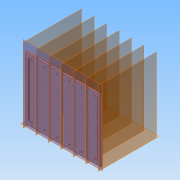
# Autodesk Inventor part: Selection_Ramp 1
Saved by Autodesk Inventor 2018.1 (Build 221171000, 171)
## iProperties
Created: 2019-02-07
Part Number: Selection_Ramp 1
Material: Wood (Oak)
Document SubType Name: Modeling
Designer: James
Density: 0.76 g/cm^3
Appearance: White Oak - Natural Medium Gloss
Author: James
Autodesk Inventor part; units mm, degrees
ref_plane "YZ Plane" through (0, 0, 0) normal (1, 0, 0) x (0, 1, 0)
ref_plane "XZ Plane" through (0, 0, 0) normal (0, 1, 0) x (-1, 0, 0)
ref_plane "XY Plane" through (0, 0, 0) normal (0, 0, 1) x (1, 0, 0)
derived "Prototype_Skeleton.ipt"
ref_plane "Ground" through (0, 0, 0) normal (0, 1, 0) x (-1, 0, 0)
ref_plane "LHS inner" through (0, 0, 0) normal (1, 0, 0) x (0, 1, 0)
ref_plane "RHS inner" through (300, 0, 0) normal (1, 0, 0) x (0, 1, 0)
ref_plane "Lane 1" through (50, 0, 0) normal (1, 0, 0) x (0, 1, 0)
ref_plane "Lane 2" through (100, 0, 0) normal (1, 0, 0) x (0, 1, 0)
ref_plane "Lane 3" through (150, 0, 0) normal (1, 0, 0) x (0, 1, 0)
ref_plane "Lane 4" through (200, 0, 0) normal (1, 0, 0) x (0, 1, 0)
ref_plane "Lane 5" through (250, 0, 0) normal (1, 0, 0) x (0, 1, 0)
ref_plane "Back" through (0, 0, 0) normal (0, 0, 1) x (1, 0, 0)
sketch "Sketch1" plane through (0, 0, 0) normal (0, 1, 0) x (-1, 0, 0)
  line L0 (-300, -50) -> (-300, 300) projected
  line L1 (0, -50) -> (0, 300) projected
  line L2 (-360, 0) -> (60, 0) projected
  line L3 (0, 0) -> (-300, 0)
  line L4 (-300, 0) -> (-300, 250)
  line L5 (-300, 250) -> (0, 250)
  line L6 (0, 250) -> (0, 0)
  dimension "d1" = 250
  constraints: 8 end point, 2 parallel, 1 horizontal, 1 perpendicular, 1 point on line
  measures "d1" distance of L3.end L4.end
extrude "Extrusion1" add sketch "Sketch1" along normal blind 5
sketch "Sketch2" plane through (0, 5, 0) normal (0, 1, 0) x (1, 0, 0)
  line L0 (300, 0) -> (0, 0) projected
  line L1 (0, -250) -> (300, -250) projected
  line L2 (50, 50) -> (50, -300) projected
  point P0 (25, -15)
  point P1 (25, -235)
  dimension "d4" = 15
  dimension "d5" = 15
  dimension "d6" = 220
  dimension "d7" = 25
  constraints: 1 vertical alignment
  measures "d4" distance from line of point (25, -15) L0
  measures "d5" distance from line of L1 point (25, -235)
  measures "d6" distance of point (25, -15) point (25, -235)
  measures "d7" distance from line of L2 point (25, -15)
hole "Hole1" at (25, 5, 15) at (25, 5, 235) direction (0, -1, 0) diameter 4.5 end through all clearance for "Socket Head Cap Screw" size "M4" standard "Ansi Metric M Profile"
pattern_linear "Rectangular Pattern1" count 6 spacing 50 along (1, 0, 0) of "Hole1"
ref_plane "Mid Plane" through (150, 0, 0) normal (-1, 0, 0) x (0, 0, 1)
sketch "Sketch4" plane through (0, 5, 0) normal (0, 1, 0) x (1, 0, 0)
  line L0 (0, 0) -> (0, -250) projected
  line L1 (300, 0) -> (0, 0) projected
  line L2 (0, -250) -> (300, -250) projected
  point P0 (12.5, -167.5)
  point P1 (12.5, -232.5)
  dimension "d29" = 12.5
  dimension "d30" = 65
  dimension "d40" = 17.5
  constraints: 1 vertical alignment
  measures "d29" distance from line of L0 point (12.5, -167.5)
  measures "d30" distance of point (12.5, -167.5) point (12.5, -232.5)
  measures "d40" distance from line of L2 point (12.5, -232.5)
hole "Hole3" at (12.5, 5, 167.5) at (12.5, 5, 232.5) direction (0, -1, 0) diameter 4.5 end through all clearance for "Flat Head Machine Screw" size "M4" standard "Ansi Metric M Profile"
mirror "Mirror2" about plane through (150, 0, 0) normal (-1, 0, 0) of "Hole3"
sketch "Sketch5" plane through (0, 5, 0) normal (0, 1, 0) x (1, 0, 0)
  circle A0 centre (12.5, -232.5) radius 2.25 projected
  line L0 (12.5, -232.5) -> (12.5, -17.5) construction
  line L1 (0, 0) -> (0, -250) projected
  line L2 (10.25, -232.5) -> (10.25, -17.5)
  line L3 (14.75, -17.5) -> (14.75, -232.5)
  arc A1 (10.25, -232.5) -> (14.75, -232.5) centre (12.5, -232.5) ccw
  arc A2 (14.75, -17.5) -> (10.25, -17.5) centre (12.5, -17.5) ccw
  line L4 (0, -250) -> (300, -250) projected
  line L5 (360, 0) -> (-60, 0) projected
  point P0 (12.5, -125)
  point P1 (12.5, -234.75)
  dimension "d41" = 17.5
  dimension "d42" = 17.5
  constraints: 8 end point, 5 point on circle, 4 tangent, 2 centre point, 2 parallel, 1 midpoint, 1 vertical alignment, 1 other
  measures "d41" distance from line of L0.start L4
  measures "d42" distance from line of L0.end L5
extrude "Extrusion2" cut sketch "Sketch5" against normal through all contours A0 L2 A2 L3
mirror "Mirror3" about plane through (150, 0, 0) normal (1, 0, 0) of "Extrusion2"
equation "\"d5\" = d4"
equation "\"d42\" = d41"
body "Solid1"
